Autodesk Fusion 360 part; units mm, degrees
note: some values were not read from the file. Set by a fixed rule: which face or edge a step refers to.
(part 3 of 5)
sketch "Sketch83" plane through (0, 0, 0) normal (0, -1, 0) x (1, 0, 0)
  line L0 (99.6333, 126.9) -> (110.3667, 126.9)
  line L1 (110.3667, 126.9) -> (110.3667, 121.1)
  line L2 (110.3667, 121.1) -> (99.6333, 121.1)
  line L3 (99.6333, 121.1) -> (99.6333, 126.9)
  line L4 (137, 156) -> (105, 156)
  line L5 (105, 156) -> (105, 168)
  line L6 (105, 168) -> (73, 168)
  line L7 (73, 168) -> (73, 134)
  line L8 (99.6333, 134) -> (99.6334, 134)
  line L9 (98.0333, 134) -> (98.0333, 125)
  line L10 (105, 126.9) -> (105, 121.1)
  line L11 (103.9129, 123.9) -> (108.9129, 123.9)
  line L12 (103.9129, 123.9) -> (111.9129, 123.9)
  line L13 (111.9129, 123.9) -> (132.4129, 123.9)
  line L14 (132.4129, 123.9) -> (132.4129, 152.9)
  line L15 (132.4129, 152.9) -> (111.9129, 152.9)
  line L16 (111.9129, 152.9) -> (111.9129, 123.9)
  line L17 (111.9129, 123.9) -> (111.9129, 136.9)
  line L18 (111.9129, 136.9) -> (107.9129, 136.9)
  line L19 (107.9129, 136.9) -> (111.9129, 136.9)
  line L20 (111.9129, 136.9) -> (111.9129, 152.9)
  line L21 (111.9129, 152.9) -> (107.9129, 152.9)
  line L22 (107.9129, 152.9) -> (107.9129, 136.9)
  line L23 (111.9129, 136.9) -> (132.4129, 136.9)
  line L24 (132.4129, 136.9) -> (136.4129, 136.9)
  line L25 (136.4129, 136.9) -> (132.4129, 136.9)
  line L26 (132.4129, 136.9) -> (132.4129, 152.9)
  line L27 (132.4129, 152.9) -> (136.4129, 152.9)
  line L28 (136.4129, 152.9) -> (136.4129, 136.9)
  line L29 (110.3667, 126.9) -> (111.9129, 126.9)
  line L30 (111.9129, 126.9) -> (107.9129, 126.9)
  line L31 (107.9129, 126.9) -> (107.9129, 136.9)
  line L32 (107.9129, 136.9) -> (111.9129, 136.9)
  line L33 (111.9129, 136.9) -> (111.9129, 126.9)
  line L34 (111.9129, 126.9) -> (132.4129, 126.9)
  line L35 (132.4129, 126.9) -> (136.4129, 126.9)
  line L36 (136.4129, 136.9) -> (136.4129, 126.9)
  line L37 (105, 126.9) -> (105, 123.9)
  line L38 (111.9129, 152.9) -> (113.9129, 152.9)
  line L39 (113.9129, 152.9) -> (113.9129, 155)
  line L40 (113.9129, 155) -> (111.9129, 155)
  line L41 (111.9129, 155) -> (111.9129, 152.9)
  line L42 (105, 138.9) -> (105, 133.1)
  line L43 (99.6333, 136) -> (105, 136)
  line L44 (105, 138.9) -> (105, 134)
  line L45 (105, 134) -> (97, 134)
  line L46 (97, 134) -> (76.5, 134)
  line L47 (76.5, 134) -> (76.5, 163)
  line L48 (76.5, 163) -> (97, 163)
  line L49 (97, 163) -> (97, 134)
  line L50 (97, 147) -> (101, 147)
  line L51 (101, 147) -> (97, 147)
  line L52 (97, 147) -> (97, 134)
  line L53 (97, 134) -> (101, 134)
  line L54 (101, 134) -> (101, 147)
  line L55 (97, 147) -> (76.5, 147)
  line L56 (76.5, 147) -> (72.5, 147)
  line L57 (72.5, 147) -> (76.5, 147)
  line L58 (76.5, 147) -> (76.5, 134)
  line L59 (76.5, 134) -> (72.5, 134)
  line L60 (72.5, 134) -> (72.5, 147)
  line L61 (97, 163) -> (95, 163)
  line L62 (95, 163) -> (95, 167)
  line L63 (95, 167) -> (97, 167)
  line L64 (97, 167) -> (97, 163)
  line L65 (97, 167) -> (95, 167)
  line L66 (95, 167) -> (95, 168)
  line L67 (95, 168) -> (97, 168)
  line L68 (97, 168) -> (97, 167)
  line L69 (111.9129, 155) -> (115, 155)
  line L70 (115, 155) -> (115, 156)
  line L71 (115, 156) -> (111.9129, 156)
  line L72 (111.9129, 156) -> (111.9129, 155)
  line L73 (110.3667, 133.1) -> (99.6333, 133.1)
  line L74 (99.6333, 133.1) -> (99.6333, 134)
  line L75 (99.6333, 138.9) -> (110.3667, 138.9)
  line L76 (110.3667, 138.9) -> (110.3667, 133.1)
  line L77 (98.0333, 125) -> (30, 125)
  line L78 (30, 125) -> (30, 115)
  line L79 (30, 115) -> (180, 115)
  line L80 (180, 115) -> (180, 125)
  line L81 (180, 125) -> (137, 125)
  line L82 (137, 125) -> (137, 156)
  line L83 (99.6333, 133.1) -> (105, 133.1)
  line L84 (105, 133.1) -> (105, 138.9)
  line L85 (105, 138.9) -> (99.6333, 138.9)
  line L86 (99.6333, 138.9) -> (99.6333, 133.1)
  line L87 (99.6334, 134) -> (99.6333, 136)
  line L88 (99.6333, 136) -> (99.6333, 138.9)
  line L89 (111.9129, 126.9) -> (107.9129, 126.9)
  line L90 (136.4129, 136.9) -> (137, 136.9)
  line L91 (136.4129, 126.9) -> (137, 126.9)
  line L92 (73, 134) -> (98.0333, 134)
  dimension "d705" = 5
  dimension "d706" = 8
  dimension "d707" = 20.5
  dimension "d708" = 29
  dimension "d709" = 13
  dimension "d710" = 4
  dimension "d711" = 4
  dimension "d712" = 4
  dimension "d715" = 3
  dimension "d716" = 2
  dimension "d718" = 8
  dimension "d719" = 20.5
  dimension "d720" = 29
  dimension "d721" = 4
  dimension "d722" = 13
  dimension "d723" = 4
  dimension "d724" = 2
  dimension "d753" = 2
  constraint midpoint L0 L10.start
  constraint midpoint L2 L10.end
  constraint perpendicular L10 L11
  constraint perpendicular L10 L12
  constraint horizontal L13
  constraint vertical L14
  constraint horizontal L15
  constraint vertical L16
  constraint coincident L16 L17.end
  constraint perpendicular L17 L18
  constraint horizontal L19
  constraint vertical L20
  constraint horizontal L21
  constraint vertical L22
  constraint coincident L14 L23.end
  constraint perpendicular L14 L23
  constraint perpendicular L14 L24
  constraint horizontal L25
  constraint vertical L26
  constraint horizontal L27
  constraint vertical L28
  constraint coincident L0.end L1.start
  constraint coincident L17 L29.end
  constraint horizontal L30
  constraint vertical L31
  constraint horizontal L32
  constraint vertical L33
  constraint coincident L14 L34.end
  constraint perpendicular L14 L34
  constraint perpendicular L35 L36
  constraint perpendicular L11 L37
  constraint coincident L12 L37.end
  constraint horizontal L38
  constraint vertical L39
  constraint horizontal L40
  constraint vertical L41
  constraint midpoint L42 L43.end
  constraint horizontal L46
  constraint vertical L47
  constraint horizontal L48
  constraint vertical L49
  constraint coincident L49 L50.start
  constraint perpendicular L49 L50
  constraint horizontal L51
  constraint vertical L52
  constraint horizontal L53
  constraint vertical L54
  constraint coincident L47 L55.end
  constraint perpendicular L47 L55
  constraint perpendicular L47 L56
  constraint horizontal L57
  constraint vertical L58
  constraint horizontal L59
  constraint vertical L60
  constraint horizontal L61
  constraint vertical L62
  constraint horizontal L63
  constraint vertical L64
  constraint horizontal L65
  constraint vertical L66
  constraint horizontal L67
  constraint vertical L68
  constraint coincident L6 L66.end
  constraint horizontal L69
  constraint vertical L70
  constraint horizontal L71
  constraint vertical L72
  constraint coincident L4 L70.end
  constraint horizontal L83
  constraint vertical L84
  constraint horizontal L85
  constraint vertical L86
  constraint coincident L73.end L74.start
  constraint collinear L29 L30
  constraint coincident L82 L90.end
  constraint perpendicular L82 L90
  constraint coincident L82 L91.end
  constraint perpendicular L82 L91
  measures "d705" distance of L11.start L11.end
  measures "d706" distance of L11.start L12.end
  measures "d707" distance of L12.end L13.end
  measures "d708" distance of L12.end L15.end
  measures "d709" distance of L12.end L17.end
  measures "d710" distance of L17.end L18.end
  measures "d711" distance of L23.end L24.end
  measures "d712" distance of L34.end L35.end
  measures "d715" distance of L10.start L37.end
  measures "d716" distance of L15.end L38.end
  measures "d718" distance of L44.end L45.end
  measures "d719" distance of L45.end L46.end
  measures "d720" distance of L45.end L48.end
  measures "d721" distance of L50.start L50.end
  measures "d722" distance of L45 L50
  measures "d723" distance of L55.end L56.end
  measures "d724" distance of L48.end L61.end
  measures "d753" distance of L43 L45
extrude "Extrude50" cut sketch "Sketch83" against normal blind 10 contours L0 L16 L17 L18 L19 L29 L30 L31 L32 L33 L73 L76 L89 | L1 L12 L16 L17 L29 L30 L89 | L13 L14 L16 L17 L34 | L14 L16 L17 L23 L33 L34 | L14 L15 L16 L20 L23 L26 L38 | L14 L24 L25 L35 L36 | L15 L38 L39 L40 L41 L69 | L36 L82 L90 L91 | L4 L40 L69 L70 L71 L72 bodies 5 in component "inner_adapter"
extrude "Extrude51" cut sketch "Sketch83" against normal blind 10 contours L43 L45 L53 L54 L86 L87 | L45 L49 L50 L51 L52 L53 L54 L75 L85 L86 L87 L88 L92 | L43 L54 L75 L85 L86 L88 | L46 L47 L49 L52 L55 L58 L92 | L47 L48 L49 L55 L61 | L7 L47 L56 L57 L58 L59 L92 | L48 L61 L62 L63 L64 L65 | L7 L56 L57 L59 L60 | L6 L63 L65 L66 L67 L68 bodies 5 in component "inner_adapter"
extrude "Extrude44" add sketch "Sketch81" along normal blind 10 and the other way blind 11 separate body contours L3 L4 L5 L6 L10 | L6 L7 L8 L9 L10 | L25 L27 L37 L40 L41 | L32 L37 L38 L39 L40 makes body 7 at (103.3444, 8, 138.5) makes body 8 at (106.6556, 15, 126.5)
sketch "Sketch84" plane through (100.0333, 0, 0) normal (-1, 0, 0) x (0, -1, 0)
  line L0 (-22, 133.5) -> (-1, 133.5)
  line L1 (-1, 133.5) -> (-1, 138.5)
  line L2 (-1, 138.5) -> (-22, 138.5)
  line L3 (-22, 138.5) -> (-22, 133.5)
  line L4 (-22, 138.5) -> (-16, 138.5)
  line L5 (-22, 133.5) -> (-16, 138.5)
  line L6 (-22, 133.5) -> (-22, 138.5)
  line L7 (-22, 126.5) -> (-22, 121.5)
  line L8 (-22, 121.5) -> (-16, 121.5)
  line L9 (-22, 126.5) -> (-16, 121.5)
  line L10 (0, 125) -> (0, 134)
  line L11 (0, 134) -> (-10, 134)
  line L12 (-10, 134) -> (-11, 134)
  line L13 (-11, 134) -> (-11, 125)
  line L14 (-11, 125) -> (0, 125)
  line L15 (-22, 133.5) -> (-21.5, 133.5)
  line L16 (-21.5, 133.5) -> (-21.5, 133.9167)
  line L17 (-22, 121.5) -> (-1, 121.5)
  line L18 (-22, 126.5) -> (-1, 126.5)
  line L19 (-22, 126.5) -> (-21.5, 126.5)
  line L20 (-21.5, 126.5) -> (-21.5, 126.0833)
  dimension "d731" = 6
  dimension "d732" = 6
  dimension "d948" = 0.5
  dimension "d949" = 0.5
  constraint coincident L2.end L3.start
  constraint perpendicular L3 L4
  constraint coincident L0.start L3.end
  constraint perpendicular L4 L7
  constraint perpendicular L7 L8
  constraint perpendicular L6 L15
  constraint coincident L5 L16.end
  constraint perpendicular L15 L16
  constraint collinear L8 L17
  constraint coincident L7.start L9.start
  constraint perpendicular L7 L19
  constraint coincident L9 L20.end
  constraint perpendicular L19 L20
  measures "d731" distance of L2.end L4.end
  measures "d732" distance of L7.end L8.end
  measures "d948" distance of L0.start L15.end
  measures "d949" distance of L7.start L19.end
extrude "Extrude45" cut sketch "Sketch84" against normal blind 10 contours L0 L5 L15 L16 | L2 L3 L4 L5 L6 | L7 L8 L9 L17 | L9 L18 L19 L20 bodies 8 7
sketch "Sketch85" plane through (100.0333, 0, 0) normal (-1, 0, 0) x (0, -1, 0)
  line L0 (-16, 138.5) -> (-21.5, 133.9167)
  line L1 (-21.5, 133.5) -> (-1, 133.5)
  line L2 (-1, 133.5) -> (-1, 138.5)
  line L3 (-1, 138.5) -> (-16, 138.5)
  line L4 (0, 125) -> (0, 134)
  line L5 (-3, 137.5) -> (-15, 137.5)
  line L6 (-15, 137.5) -> (-15, 134.5)
  line L7 (-15, 134.5) -> (-3, 134.5)
  line L8 (-3, 134.5) -> (-3, 137.5)
  line L9 (-10, 134) -> (-10, 147)
  line L10 (0, 134) -> (-10, 134)
  line L11 (-16, 138.5) -> (-16, 133.5)
  line L12 (-16, 136) -> (-14, 136)
  line L13 (-10, 134) -> (-11, 134)
  line L14 (-11, 134) -> (-11, 125)
  line L15 (-11, 125) -> (0, 125)
  line L16 (-21.5, 133.9167) -> (-21.5, 133.5)
  dimension "d735" = 2
  dimension "d736" = 5
  dimension "d754" = 3
  constraint horizontal L5
  constraint vertical L6
  constraint horizontal L7
  constraint vertical L8
  constraint coincident L0.start L3.end
  constraint coincident L1 L11.end
  constraint perpendicular L1 L11
  constraint midpoint L11 L12.start
  constraint perpendicular L11 L12
  constraint midpoint L6 L12
  measures "d735" distance of L2 L8
  measures "d736" distance of L6 L9
  measures "d754" distance of L5 L7
extrude "Extrude46'" cut sketch "Sketch85" against normal blind 8 contours L5 L6 L7 L9 | L5 L7 L8 L9 bodies 7
copy_body "Body->Comp6" bodies 7 removing the originals makes body 9 in component "Pins"
copy_body "Body->Comp7" bodies 8 removing the originals makes body 10 in component "Component"
copy_body "CutPasteBodies1" bodies 10 removing the originals makes body 11 in component "Pins"
sketch "Sketch86" plane through (0, 0, 0) normal (0, -1, 0) x (1, 0, 0)
  line L0 (97, 168) -> (97, 147)
  line L1 (97, 147) -> (101, 147)
  line L2 (101, 147) -> (101, 138.9)
  line L3 (111.9129, 136.9) -> (111.9129, 156)
  line L4 (111.9129, 156) -> (105, 156)
  line L5 (105, 156) -> (105, 168)
  line L6 (105, 168) -> (97, 168)
  circle A0 centre (105, 143) radius 2
  line L7 (98.0333, 134) -> (98.0333, 125)
  line L8 (132.4129, 126.9) -> (132.4129, 123.9)
  line L9 (132.4129, 123.9) -> (110.3667, 123.9)
  line L10 (110.3667, 123.9) -> (110.3667, 121.1)
  line L11 (110.3667, 121.1) -> (99.6333, 121.1)
  line L12 (99.6333, 121.1) -> (99.6333, 126.9)
  line L13 (99.6333, 126.9) -> (107.9129, 126.9)
  line L14 (101, 138.9) -> (110.3667, 138.9)
  line L15 (110.3667, 138.9) -> (110.3667, 136.9)
  line L16 (99.6333, 134) -> (98.0333, 134)
  line L17 (98.0333, 125) -> (30, 125)
  line L18 (30, 125) -> (30, 115)
  line L19 (30, 115) -> (180, 115)
  line L20 (180, 115) -> (180, 125)
  line L21 (180, 125) -> (137, 125)
  line L22 (137, 125) -> (137, 126.9)
  line L23 (137, 126.9) -> (132.4129, 126.9)
  line L24 (107.9129, 133.1) -> (99.6333, 133.1)
  line L25 (99.6333, 133.1) -> (99.6333, 134)
  line L26 (110.3667, 136.9) -> (111.9129, 136.9)
  line L27 (107.9129, 126.9) -> (107.9129, 133.1)
  circle A1 centre (101, 164) radius 2
  dimension "d740" = 4
  dimension "d929" = 4
  dimension "d930" = 4
  dimension "d931" = 4
  measures "d740" diameter of A0
  measures "d929" diameter of A1
  measures "d930" distance of L6 A1.centre
  measures "d931" distance of L0 A1.centre
extrude "Extrude52" cut sketch "Sketch86" against normal blind 8 contours A0 | A1 bodies 5 in component "inner_adapter"
sketch "Sketch87" plane through (101, 0, 0) normal (-1, 0, 0) x (0, -1, 0)
  line L0 (0, 138.9) -> (0, 147)
  line L1 (0, 147) -> (-10, 147)
  line L2 (-10, 147) -> (-10, 138.9)
  line L3 (-8, 145) -> (-8, 141)
  line L4 (0, 145) -> (0, 141)
  line L5 (-8, 146.5) -> (-4.9, 146.5)
  line L6 (-4.9, 146.5) -> (-4.9, 139.5)
  line L7 (-4.9, 139.5) -> (-8, 139.5)
  line L8 (-8, 139.5) -> (-8, 146.5)
  line L9 (-10, 138.9) -> (0, 138.9)
  dimension "d745" = 3.1
  dimension "d746" = 7
  constraint horizontal L5
  constraint vertical L6
  constraint horizontal L7
  constraint vertical L8
  constraint midpoint L3 L8
  measures "d745" distance of L5.start L5.end
  measures "d746" distance of L5.start L7.end
sketch "Sketch102" plane through (105, 0, 0) normal (1, 0, 0) x (0, 1, 0)
  line L0 (11, 156) -> (11, 168)
  line L1 (11, 168) -> (0, 168)
  line L2 (0, 168) -> (0, 156)
  line L3 (0, 156) -> (11, 156)
  line L4 (8, 162) -> (8, 166)
  line L5 (0, 162) -> (0, 166)
  line L6 (8, 164) -> (8, 160.5)
  line L7 (8, 160.5) -> (4.9, 160.5)
  line L8 (4.9, 160.5) -> (4.9, 167.5)
  line L9 (4.9, 167.5) -> (8, 167.5)
  line L10 (8, 167.5) -> (8, 160.5)
  dimension "d932" = 3.5
  dimension "d933" = 3.1
  dimension "d934" = 7
  constraint midpoint L4 L6.start
  constraint parallel L4 L6
  constraint horizontal L7
  constraint vertical L8
  constraint horizontal L9
  constraint vertical L10
  measures "d932" distance of L6.start L6.end
  measures "d933" distance of L6.end L7.end
  measures "d934" distance of L6.end L9.end
extrude "Extrude60" cut sketch "Sketch102" against normal blind 8 contours L4 L6 L7 L8 L9 L10 bodies 5 in component "inner_adapter"
extrude "Extrude53" cut sketch "Sketch87" against normal blind 8 contours L3 L5 L6 L7 L8 bodies 5 in component "inner_adapter"
sketch "Sketch89" plane through (109.9667, 0, 0) normal (1, 0, 0) x (0, 1, 0)
  line L0 (16, 121.5) -> (21.5, 126.0833)
  line L1 (21.5, 126.5) -> (1, 126.5)
  line L2 (1, 126.5) -> (1, 121.5)
  line L3 (1, 121.5) -> (16, 121.5)
  line L4 (16, 121.5) -> (16, 126.5)
  line L5 (16, 124) -> (14, 124)
  line L6 (3, 125.5) -> (15, 125.5)
  line L7 (15, 125.5) -> (15, 122.5)
  line L8 (15, 122.5) -> (3, 122.5)
  line L9 (3, 122.5) -> (3, 125.5)
  line L10 (3, 134.5) -> (3, 137.5)
  line L11 (3, 137.5) -> (15, 137.5)
  line L12 (15, 137.5) -> (15, 134.5)
  line L13 (15, 134.5) -> (3, 134.5)
  line L14 (3, 137.5) -> (3, 121.5)
  line L15 (15, 137.5) -> (15, 121)
  line L16 (21.5, 126.0833) -> (21.5, 126.5)
  dimension "d758" = 3
  constraint coincident L0.start L3.end
  constraint coincident L1 L4.end
  constraint perpendicular L1 L4
  constraint midpoint L4 L5.start
  constraint perpendicular L4 L5
  constraint horizontal L6
  constraint vertical L7
  constraint horizontal L8
  constraint vertical L9
  constraint midpoint L5 L7
  constraint coincident L10.end L11.start
  constraint perpendicular L11 L14
  constraint coincident L11.end L12.start
  constraint perpendicular L11 L15
  constraint collinear L7 L15
  constraint collinear L9 L14
  measures "d758" distance of L6 L8
extrude "Extrude1'''" cut sketch "Sketch89" against normal blind 8 contours L6 L7 L8 L9 L14 L15 bodies 11 in component "Pins"
sketch "Sketch126" plane through (0, 16, 0) normal (0, 1, 0) x (-1, 0, 0)
  line L0 (-135, 115) -> (-75, 115)
  line L1 (-75, 115) -> (-75, 205)
  line L2 (-75, 205) -> (-135, 205)
  line L3 (-135, 205) -> (-135, 115)
  line L4 (-110.3667, 138.9) -> (-99.6333, 138.9)
  line L5 (-99.6333, 138.9) -> (-99.6333, 133.1)
  line L6 (-99.6333, 133.1) -> (-110.3667, 133.1)
  line L7 (-110.3667, 133.1) -> (-110.3667, 138.9)
  line L8 (-110.3667, 121.1) -> (-110.3667, 126.9)
  line L9 (-110.3667, 126.9) -> (-99.6333, 126.9)
  line L10 (-99.6333, 126.9) -> (-99.6333, 121.1)
  line L11 (-99.6333, 121.1) -> (-110.3667, 121.1)
  line L12 (-115, 131.5) -> (-95, 131.5)
  line L13 (-95, 131.5) -> (-95, 128.5)
  line L14 (-95, 128.5) -> (-115, 128.5)
  line L15 (-115, 128.5) -> (-115, 131.5)
  line L16 (-105, 126.9) -> (-105, 128.5)
  dimension "d1103" = 20
  dimension "d1104" = 3
  dimension "d1105" = 1.6
  constraint horizontal L12
  constraint vertical L13
  constraint horizontal L14
  constraint vertical L15
  constraint midpoint L9 L16.start
  constraint midpoint L14 L16.end
  constraint parallel L8 L16
  measures "d1103" distance of L12.start L12.end
  measures "d1104" distance of L12.start L14.end
  measures "d1105" distance of L16.start L16.end
extrude "Extrude77" cut sketch "Sketch126" against normal blind 3 contours L12 L13 L14 L15 bodies 5 in component "inner_adapter"
sketch "Sketch127" plane through (0, 18, 0) normal (0, -1, 0) x (1, 0, 0)
  line L0 (75, 127.5) -> (135, 127.5)
  line L1 (135, 127.5) -> (135, 132.5)
  line L2 (135, 132.5) -> (75, 132.5)
  line L3 (75, 132.5) -> (75, 127.5)
  line L4 (95, 131.5) -> (115, 131.5)
  line L5 (115, 131.5) -> (95, 131.5)
  line L6 (115, 131.5) -> (95, 131.5)
  line L7 (95, 128.5) -> (115, 128.5)
  line L8 (95, 131.5) -> (95, 128.5)
  line L9 (115, 128.5) -> (115, 131.5)
extrude "Extrude10" cut sketch "Sketch127" against normal blind 3 contours L4 L5 L6 L7 L8 L9 bodies 6 in component "Flap"
sketch "Sketch95" plane through (0, 0, 0) normal (0, -1, 0) x (1, 0, 0)
  circle A0 centre (105, 143) radius 2
  line L0 (97, 168) -> (97, 147)
  line L1 (97, 147) -> (101, 147)
  line L2 (101, 147) -> (101, 138.9)
  line L3 (111.9129, 136.9) -> (111.9129, 156)
  line L4 (111.9129, 156) -> (105, 156)
  line L5 (105, 156) -> (105, 168)
  line L6 (105, 168) -> (97, 168)
  line L7 (95, 163) -> (95, 168)
  line L8 (95, 168) -> (73, 168)
  line L9 (73, 168) -> (73, 147)
  line L10 (73, 147) -> (76.5, 147)
  line L11 (76.5, 147) -> (76.5, 163)
  line L12 (76.5, 163) -> (95, 163)
  line L13 (98.0333, 134) -> (98.0333, 125)
  line L14 (132.4129, 126.9) -> (132.4129, 123.9)
  line L15 (132.4129, 123.9) -> (110.3667, 123.9)
  line L16 (110.3667, 123.9) -> (110.3667, 121.1)
  line L17 (110.3667, 121.1) -> (99.6333, 121.1)
  line L18 (99.6333, 121.1) -> (99.6333, 126.9)
  line L19 (99.6333, 126.9) -> (107.9129, 126.9)
  line L20 (73, 168) -> (137, 168)
  line L21 (137, 168) -> (137, 125)
  line L22 (137, 125) -> (73, 125)
  line L23 (73, 125) -> (73, 168)
  circle A1 centre (105, 143) radius 2
  line L24 (110.3667, 138.9) -> (110.3667, 136.9)
  line L25 (101, 138.9) -> (110.3667, 138.9)
  line L26 (110.3667, 123.9) -> (110.3667, 126.9)
  line L27 (110.3667, 138.9) -> (94.3667, 138.9)
  line L28 (94.3667, 138.9) -> (94.3667, 133.1)
  line L29 (94.3667, 133.1) -> (110.3667, 133.1)
  line L30 (110.3667, 133.1) -> (110.3667, 138.9)
  line L31 (110.3667, 126.9) -> (99.6333, 126.9)
  line L32 (99.6333, 126.9) -> (99.6333, 121.1)
  line L33 (99.6333, 121.1) -> (110.3667, 121.1)
  line L34 (110.3667, 121.1) -> (110.3667, 126.9)
  line L35 (137, 125) -> (99.6333, 125)
  line L36 (99.6333, 125) -> (99.6333, 121.1)
  line L37 (99.6333, 121.1) -> (137, 121.1)
  line L38 (137, 121.1) -> (137, 125)
  line L39 (137, 121.1) -> (73, 121.1)
  line L40 (73, 121.1) -> (73, 125)
  line L41 (73, 125) -> (137, 125)
  line L42 (137, 125) -> (137, 121.1)
  line L43 (73, 121.1) -> (137, 121.1)
  line L44 (137, 121.1) -> (137, 118.1)
  line L45 (137, 118.1) -> (73, 118.1)
  line L46 (73, 118.1) -> (73, 121.1)
  line L47 (101, 138.9) -> (110.3667, 138.9)
  line L48 (110.3667, 138.9) -> (110.3667, 136.9)
  line L49 (99.6333, 134) -> (98.0333, 134)
  line L50 (98.0333, 125) -> (30, 125)
  line L51 (30, 125) -> (30, 115)
  line L52 (30, 115) -> (180, 115)
  line L53 (180, 115) -> (180, 125)
  line L54 (180, 125) -> (137, 125)
  line L55 (137, 125) -> (137, 126.9)
  line L56 (137, 126.9) -> (132.4129, 126.9)
  line L57 (107.9129, 133.1) -> (99.6333, 133.1)
  line L58 (99.6333, 133.1) -> (99.6333, 134)
  line L59 (137, 126.9) -> (132.4129, 126.9)
  line L60 (110.3667, 136.9) -> (111.9129, 136.9)
  line L61 (107.9129, 126.9) -> (107.9129, 133.1)
  circle A2 centre (101, 164) radius 2
  line L62 (99.6333, 126.9) -> (115.6333, 126.9)
  line L63 (115.6333, 126.9) -> (115.6333, 121.1)
  line L64 (115.6333, 121.1) -> (99.6333, 121.1)
  line L65 (99.6333, 121.1) -> (99.6333, 126.9)
  line L66 (95, 168) -> (95, 170)
  line L67 (95, 170) -> (71, 170)
  line L68 (71, 170) -> (71, 147)
  line L69 (71, 147) -> (73, 147)
  line L70 (137, 156) -> (115, 156)
  line L71 (137, 156) -> (115, 156)
  line L72 (115, 156) -> (115, 158)
  line L73 (115, 158) -> (137, 158)
  line L74 (137, 158) -> (137, 156)
  line L75 (137, 158) -> (139, 158)
  line L76 (139, 158) -> (139, 125)
  line L77 (93.8667, 132.6) -> (110.8667, 132.6)
  line L78 (110.8667, 132.6) -> (110.8667, 139.4)
  line L79 (110.8667, 139.4) -> (93.8667, 139.4)
  line L80 (93.8667, 139.4) -> (93.8667, 132.6)
  line L81 (99.1333, 127.4) -> (116.1333, 127.4)
  line L82 (116.1333, 127.4) -> (116.1333, 120.6)
  line L83 (116.1333, 120.6) -> (99.1333, 120.6)
  line L84 (99.1333, 120.6) -> (99.1333, 127.4)
  point P0 (107.9129, 126.9)
  dimension "d873" = 3
  dimension "d945" = 16
  dimension "d946" = 16
  dimension "d969" = 2
  dimension "d970" = 24
  dimension "d971" = 2
  dimension "d972" = 2
  dimension "d977" = 2
  dimension "d1044" = 0.5
  dimension "d1045" = -0.5
  constraint horizontal L20
  constraint vertical L21
  constraint horizontal L22
  constraint vertical L23
  constraint coincident L8.end L9.start
  constraint horizontal L27
  constraint vertical L28
  constraint horizontal L29
  constraint vertical L30
  constraint coincident L24.start L25.end
  constraint horizontal L31
  constraint vertical L32
  constraint horizontal L33
  constraint vertical L34
  constraint coincident L17.end L18.start
  constraint coincident L26.end L31.start
  constraint horizontal L35
  constraint vertical L36
  constraint horizontal L37
  constraint vertical L38
  constraint horizontal L39
  constraint vertical L40
  constraint horizontal L41
  constraint vertical L42
  constraint horizontal L43
  constraint vertical L44
  constraint horizontal L45
  constraint vertical L46
  constraint horizontal L62
  constraint vertical L63
  constraint horizontal L64
  constraint vertical L65
  constraint coincident L7.end L8.start
  constraint perpendicular L8 L66
  constraint perpendicular L66 L67
  constraint perpendicular L67 L68
  constraint perpendicular L23 L69
  constraint horizontal L71
  constraint vertical L72
  constraint horizontal L73
  constraint vertical L74
  constraint coincident L70.start L71.start
  constraint perpendicular L21 L75
  constraint coincident L54 L76.end
  constraint perpendicular L54 L76
  measures "d873" distance of L39.end L45.end
  measures "d945" distance of L24.start L27.end
  measures "d946" distance of L18.end L62.end
  measures "d969" distance of L7.end L66.end
  measures "d970" distance of L66.end L67.end
  measures "d971" distance of L68.end L9.end
  measures "d972" distance of L70.start L73.end
  measures "d977" distance of L73.end L75.end
extrude "Extrude47'" add sketch "Sketch95" along normal blind 5 separate body contours L0 L1 L2 L3 L4 L5 L6 L20 L60 L78 L79 | L0 L1 L2 L7 L10 L11 L12 L13 L20 L22 L23 L41 L50 L77 L79 L80 | L3 L4 L5 L14 L20 L21 L22 L35 L41 L56 L59 L60 L61 L70 L71 L72 L73 L77 L78 L81 L82 | L7 L8 L9 L10 L11 L12 L20 L23 | L8 L9 L20 L23 L66 L67 L68 L69 | L21 L54 L55 L74 L75 L76 | L21 L70 L71 L72 L73 L74 | L22 L39 L40 L41 L43 L50 L84 | L14 L21 L22 L35 L41 L55 L56 L59 | L13 L22 L41 L61 L77 L81 L84 | L37 L39 L43 L44 L45 L46 L82 L83 L84 | L14 L15 L22 L35 L37 L38 L39 L41 L42 L43 L82 | L14 L15 L22 L35 L41 L82 makes body 12
extrude "Extrude59'" add sketch "Sketch95" against normal blind 11 contours L8 L9 L20 L23 L66 L67 L68 L69 | L21 L54 L55 L74 L75 L76 | L21 L70 L71 L72 L73 L74 bodies 12
sketch "Sketch96" plane through (0, -5, 0) normal (0, -1, 0) x (1, 0, 0)
  circle A0 centre (105, 143) radius 2
  line L0 (73, 118.1) -> (137, 118.1)
  line L1 (137, 118.1) -> (137, 125)
  line L2 (137, 168) -> (95, 168)
  line L3 (73, 147) -> (73, 118.1)
  line L4 (94.3667, 138.9) -> (94.3667, 139.9)
  line L5 (94.3667, 139.9) -> (93.3667, 139.9)
  line L6 (115.6333, 121.1) -> (116.6333, 121.1017)
  line L7 (116.6333, 121.1017) -> (116.6351, 120.1017)
  line L8 (116.6351, 120.1017) -> (93.3667, 120.1017)
  line L9 (93.3667, 120.1017) -> (93.3667, 139.9)
  line L10 (93.3667, 139.9) -> (116.6351, 139.9)
  line L11 (116.6351, 139.9) -> (116.6351, 120.1017)
  line L12 (94.3667, 133.1) -> (94.3667, 132.1)
  line L13 (115.6333, 126.9) -> (115.6333, 127.9)
  line L14 (116.6351, 127.9) -> (93.3667, 127.9)
  line L15 (93.3667, 132.1) -> (116.6351, 132.1)
  circle A1 centre (105.0009, 136) radius 2.1
  line L16 (105.0009, 139.9) -> (105.0009, 132.1)
  line L17 (105.0009, 127.9) -> (105.0009, 120.1017)
  circle A2 centre (105.0009, 124.0009) radius 2.1
  circle A3 centre (101, 164) radius 2
  line L18 (95, 168) -> (95, 170)
  line L19 (95, 170) -> (71, 170)
  line L20 (71, 170) -> (71, 147)
  line L21 (71, 147) -> (73, 147)
  line L22 (137, 125) -> (139, 125)
  line L23 (139, 125) -> (139, 158)
  line L24 (139, 158) -> (137, 158)
  line L25 (137, 158) -> (137, 168)
  line L26 (93.8667, 132.6) -> (93.8667, 139.4)
  line L27 (93.8667, 139.4) -> (110.8667, 139.4)
  line L28 (110.8667, 139.4) -> (110.8667, 132.6)
  line L29 (110.8667, 132.6) -> (93.8667, 132.6)
  line L30 (116.1333, 120.6) -> (99.1333, 120.6)
  line L31 (99.1333, 120.6) -> (99.1333, 127.4)
  line L32 (99.1333, 127.4) -> (116.1333, 127.4)
  line L33 (116.1333, 127.4) -> (116.1333, 120.6)
  dimension "d876" = 1
  dimension "d877" = 1
  dimension "d878" = 1
  dimension "d879" = 1
  dimension "d880" = 1
  dimension "d881" = 1
  dimension "d882" = 4.2
  dimension "d883" = 4.2
  constraint perpendicular L4 L5
  constraint perpendicular L6 L7
  constraint horizontal L8
  constraint vertical L9
  constraint horizontal L10
  constraint vertical L11
  constraint coincident L11 L14.start
  constraint coincident L9 L14.end
  constraint perpendicular L9 L14
  constraint coincident L9 L15.start
  constraint coincident L11 L15.end
  constraint perpendicular L11 L15
  constraint coincident L12.end L15
  constraint coincident L13.end L14
  constraint midpoint L10 L16.start
  constraint midpoint L15 L16.end
  constraint midpoint A1.centre L16
  constraint midpoint L14 L17.start
  constraint midpoint L8 L17.end
  constraint midpoint L17 A2.centre
  measures "d876" distance of L4.start L4.end
  measures "d877" distance of L4.end L5.end
  measures "d878" distance of L6.start L6.end
  measures "d879" distance of L6.end L7.end
  measures "d880" distance of L12.start L12.end
  measures "d881" distance of L13.start L13.end
  measures "d882" diameter of A1
  measures "d883" diameter of A2
extrude "Extrude48'" add sketch "Sketch96" along normal blind 9 contours L4 L5 L9 L10 L12 L15 L26 L27 L29 | A1 L16 L26 L27 L29 | L4 L10 L16 L27 | A1 L16 L27 L28 L29 | L10 L11 L15 L16 L27 L28 L29 | L9 L11 L14 L15 | L12 L15 L16 L29 | L8 L9 L14 L17 L30 L31 L32 | L13 L14 L17 L32 | L6 L11 L13 L14 L32 L33 | L6 L7 L8 L11 L17 L30 L33 | L17 A2 L30 L32 L33 | L17 A2 L30 L31 L32 bodies 12
extrude "Extrude49'" add sketch "Sketch96" along normal blind 2 from surface at 9 contours L4 L5 L9 L10 L12 L15 L26 L27 L29 | A1 L16 L26 L27 L29 | L4 L10 L16 L27 | A1 L16 L27 L28 L29 | L10 L11 L15 L16 L27 L28 L29 | A1 L16 | A1 L16 | L9 L11 L14 L15 | L12 L15 L16 L29 | L8 L9 L14 L17 L30 L31 L32 | L13 L14 L17 L32 | L6 L11 L13 L14 L32 L33 | L6 L7 L8 L11 L17 L30 L33 | L17 A2 L30 L32 L33 | L17 A2 L30 L31 L32 | L17 A2 | L17 A2 bodies 12
copy_body "Body->Comp8" bodies 12 removing the originals makes body 13 in component "Mechanism_backstop"
sketch "Skizze97" plane through (0, 0, 125) normal (0, 0, 1) x (-1, 0, 0)
  line L0 (-21.3369, -104.8) -> (-24.8369, -104.8)
  line L1 (-24.8369, -104.8) -> (-24.8369, -99.2)
  line L2 (-24.8369, -99.2) -> (-21.3369, -99.2)
  line L3 (-21.3369, -99.2) -> (-21.3369, -104.8)
  line L4 (-185.1631, -104.8) -> (-188.6631, -104.8)
  line L5 (-188.6631, -104.8) -> (-188.6631, -99.2)
  line L6 (-188.6631, -99.2) -> (-185.1631, -99.2)
  line L7 (-185.1631, -99.2) -> (-185.1631, -104.8)
  circle A0 centre (-11, -70) radius 2
  circle A1 centre (-199, -70) radius 2
  circle A2 centre (-11, -140) radius 2
  circle A3 centre (-199, -140) radius 2
  circle A4 centre (-199, -35) radius 3.5
  circle A5 centre (-11, -35) radius 3.5
  circle A6 centre (-199, -175) radius 3.5
  circle A7 centre (-11, -175) radius 3.5
  arc A8 (-180, 0) -> (-210, -30) centre (-180, -30) ccw
  line L8 (-210, -30) -> (-210, -180)
  arc A9 (-210, -180) -> (-180, -210) centre (-180, -180) ccw
  line L9 (-180, -210) -> (-30, -210)
  arc A10 (-30, -210) -> (0, -180) centre (-30, -180) ccw
  line L10 (0, -180) -> (0, -30)
  arc A11 (0, -30) -> (-30, 0) centre (-30, -30) ccw
  line L11 (-137, 0) -> (-180, 0)
  line L12 (-98.0333, -11) -> (-75, -11)
  spline S0 degree 3 poles (-75, -11) (-73.6669, -11) (-72.3215, -11.1868) (-70.7827, -11.5209) (-69.7039, -11.7551) (-68.5449, -12.0678) (-67.3101, -12.4666) (-63.5716, -13.6741) (-59.3264, -15.5672) (-54.921, -17.8316) (-52.6617, -18.993) (-50.3688, -20.252) (-48.1137, -21.5656) (-43.134, -24.4661) (-38.3659, -27.5905) (-34.4467, -30.5403) (-31.6285, -32.6614) (-29.2725, -34.6734) (-27.4088, -36.5974) (-26.9392, -37.0821) (-26.4696, -37.5669) (-26, -38.0516) knots 0 0 0 0 0.068385 0.068385 0.068385 0.116327 0.116327 0.116327 0.262353 0.262353 0.262353 0.337245 0.337245 0.337245 0.502934 0.502934 0.502934 0.621914 0.621914 0.621914 0.656812 0.656812 0.656812 0.656812
  line L13 (-26, -38.0516) -> (-26, -157.5)
  line L14 (-26, -157.5) -> (-12.5, -157.5)
  line L15 (-18, -160.5) -> (-18, -186.5)
  line L16 (-18, -186.5) -> (-25, -186.5)
  line L17 (-25, -186.5) -> (-25, -160.5)
  line L18 (-26, -183) -> (-101.02, -183)
  ellipse E0 centre (-105, -188.2858) end of major axis (-105, -180.5592) minor radius 5.4567 (-108.98, -183) -> (-101.02, -183) ccw
  line L19 (-184, -183) -> (-184, -160.5)
  line L20 (-185, -160.5) -> (-185, -186.5)
  line L21 (-185, -186.5) -> (-192, -186.5)
  line L22 (-192, -186.5) -> (-192, -160.5)
  spline S1 degree 3 poles (-184, -38.0508) (-183.53, -37.5659) (-183.0599, -37.0811) (-182.5899, -36.5963) (-180.4883, -34.4285) (-177.7611, -32.1455) (-174.4691, -29.7357) (-169.3238, -25.9693) (-162.8741, -21.9475) (-156.519, -18.5779) (-152.2041, -16.29) (-147.9761, -14.3309) (-144.2124, -12.9853) (-141.9329, -12.1703) (-139.8769, -11.6068) (-138.0391, -11.287) (-137.6862, -11.2256) (-137.3408, -11.1732) (-137, -11.1307) knots -0.65681 -0.65681 -0.65681 -0.65681 -0.621923 -0.621923 -0.621923 -0.48793 -0.48793 -0.48793 -0.278155 -0.278155 -0.278155 -0.135918 -0.135918 -0.135918 -0.050335 -0.050335 -0.050335 -0.033901 -0.033901 -0.033901 -0.033901
  line L23 (-116.6351, 5) -> (-93.3667, 5)
  line L24 (-93.3667, 5) -> (-93.3667, 16)
  line L25 (-93.3667, 16) -> (-116.6351, 16)
  line L26 (-116.6351, 16) -> (-116.6351, 5)
  line L27 (-137, 0) -> (-95, 0)
  line L28 (-95, 5) -> (-137, 5)
  line L29 (-137, 5) -> (-137, 0)
  arc A12 (-180, -5) -> (-205, -30) centre (-180, -30) ccw
  line L30 (-205, -30) -> (-205, -180)
  arc A13 (-205, -180) -> (-180, -205) centre (-180, -180) ccw
  line L31 (-180, -205) -> (-30, -205)
  arc A14 (-30, -205) -> (-5, -180) centre (-30, -180) ccw
  line L32 (-5, -180) -> (-5, -30)
  arc A15 (-5, -30) -> (-30, -5) centre (-30, -30) ccw
  line L33 (-93.3667, 18) -> (-116.6351, 18)
  line L34 (-116.6351, 18) -> (-180, -5)
  line L35 (-93.3667, 18) -> (-30, -5)
  line L36 (-93.3667, 23) -> (-116.6351, 23)
  line L37 (-116.6351, 23) -> (-180, 0)
  line L38 (-180, -210) -> (-30, -210)
  arc A16 (-30, -210) -> (0, -180) centre (-30, -180) ccw
  line L39 (0, -180) -> (0, -30)
  arc A17 (0, -30) -> (-30, 0) centre (-30, -30) ccw
  arc A18 (-180, 0) -> (-210, -30) centre (-180, -30) ccw
  line L40 (-210, -30) -> (-210, -180)
  arc A19 (-210, -180) -> (-180, -210) centre (-180, -180) ccw
  line L41 (-199, -140) -> (-190, -140)
  line L42 (-199, -140) -> (-199, -150)
  line L43 (-199, -150) -> (-205, -150)
  line L44 (-199, -70) -> (-190, -70)
  line L45 (-199, -70) -> (-199, -50)
  line L46 (-199, -50) -> (-205, -50)
  line L47 (-190, -140) -> (-190, -70)
  line L48 (-105, -191.1402) -> (-105, -26.9364)
  line L49 (-199, -150) -> (-190, -150)
  line L50 (-190, -150) -> (-190, -140)
  line L51 (-190, -140) -> (-199, -140)
  line L52 (-199, -140) -> (-199, -150)
  line L53 (-199, -145) -> (-205, -145)
  line L54 (-199, -145) -> (-195, -145)
  line L55 (-195, -145) -> (-195, -140)
  line L56 (-195, -140) -> (-195, -71.0732)
  line L57 (-202.2329, -55) -> (-205, -55)
  line L58 (-11, -150) -> (-5, -150)
  line L59 (-11, -150) -> (-20, -150)
  line L60 (-11, -145) -> (-5, -145)
  line L61 (-11, -145) -> (-15, -145)
  line L62 (-15, -145) -> (-15, -140)
  line L63 (-20, -150) -> (-20, -140)
  line L64 (-15, -140) -> (-15, -71.0732)
  line L65 (-20, -140) -> (-20, -70)
  line L66 (-7.7671, -55) -> (-5, -55)
  line L67 (-11, -50) -> (-5, -50)
  line L68 (-205, -145) -> (-210, -145)
  line L69 (-205, -55) -> (-210, -55)
  line L70 (-5, -55) -> (0, -55)
  line L71 (-5, -145) -> (0, -145)
  line L72 (-20, -70) -> (-20, -50)
  line L73 (-20, -50) -> (-11, -50)
  line L74 (-15, -71.0732) -> (-15, -55)
  line L75 (-15, -55) -> (-7.7671, -55)
  line L76 (-190, -50) -> (-199, -50)
  line L77 (-195, -55) -> (-202.2329, -55)
  line L78 (-195, -71.0732) -> (-195, -55)
  line L79 (-190, -70) -> (-190, -50)
  line L80 (-137, -11.1307) -> (-137, 0)
  line L81 (-98.0333, 0) -> (-98.0333, -11)
  line L82 (-197.5, -157.5) -> (-184, -157.5)
  line L83 (-184, -157.5) -> (-184, -38.0508)
  line L84 (-93.3667, 23) -> (-30, 0)
  line L85 (-95, 0) -> (-95, 5)
  line L86 (-108.98, -183) -> (-184, -183)
  line L87 (-12.5, -157.5) -> (-12.5, -162.5)
  line L88 (-197.5, -162.5) -> (-197.5, -157.5)
  line L89 (-196.5, -162.5) -> (-197.5, -162.5)
  line L90 (-13.5, -160.5) -> (-18, -160.5)
  line L91 (-26, -160.5) -> (-26, -183)
  line L92 (-184, -160.5) -> (-185, -160.5)
  line L93 (-12.5, -162.5) -> (-13.5, -162.5)
  line L94 (-13.5, -162.5) -> (-13.5, -160.5)
  line L95 (-25, -160.5) -> (-26, -160.5)
  line L96 (-192, -160.5) -> (-196.5, -160.5)
  line L97 (-196.5, -160.5) -> (-196.5, -162.5)
  line L98 (-30, 0) -> (-98.0333, 0)
  dimension "d889" = -5
  dimension "d890" = 2
  dimension "d891" = 7
  dimension "d892" = 9
  dimension "d893" = 10
  dimension "d894" = 9
  dimension "d895" = 20
  constraint coincident A8.start L11.end
  constraint coincident A3.centre L41.start
  constraint horizontal L41
  constraint perpendicular L41 L42
  constraint coincident L30 L43.end
  constraint perpendicular L30 L43
  constraint coincident A1.centre L44.start
  constraint horizontal L44
  constraint perpendicular L44 L45
  constraint coincident L30 L46.end
  constraint perpendicular L30 L46
  constraint horizontal L49
  constraint vertical L50
  constraint horizontal L51
  constraint vertical L52
  constraint symmetric L41.end L48 L63.end
  constraint symmetric L42.end L48 L58.start
  constraint symmetric L43.end L48 L58.end
  constraint symmetric L44.end L48 L65.end
  constraint symmetric L45.end L48 L67.start
  constraint symmetric L46.end L48 L67.end
  constraint symmetric L48 L49.end L59.end
  constraint symmetric L48 L53.start L60.start
  constraint symmetric L48 L53.end L60.end
  constraint symmetric L48 L54.end L61.end
  constraint symmetric L48 L55.end L62.end
  constraint symmetric L48 L56.end L64.end
  constraint symmetric L48 L57.start L66.start
  constraint symmetric L48 L57.end L66.end
  constraint perpendicular L30 L68
  constraint coincident L8 L69.end
  constraint perpendicular L8 L69
  constraint coincident L39 L70.end
  constraint perpendicular L39 L70
  constraint coincident L10 L71.end
  constraint perpendicular L10 L71
  constraint perpendicular L67 L72
  constraint perpendicular L32 L73
  constraint parallel L64 L74
  constraint symmetric L48 L64.end L56.end
  constraint symmetric L48 L65.end L44.end
  constraint symmetric L48 L66.start L57.start
  constraint symmetric L48 L67.start L45.end
  constraint symmetric L48 L72.end L76.start
  constraint symmetric L48 L74.end L77.start
  constraint coincident A11.end A17.end
  measures "d892" distance of A3.centre L41.end
  measures "d893" distance of A3.centre L42.end
  measures "d894" distance of A1.centre L44.end
  measures "d895" distance of A1.centre L45.end
sketch "Sketch103" plane through (0, 1, 0) normal (0, -1, 0) x (1, 0, 0)
  line L0 (109.9667, 133.5) -> (109.9667, 138.5)
  line L1 (109.9667, 138.5) -> (100.0333, 138.5)
  line L2 (100.0333, 138.5) -> (100.0333, 133.5)
  line L3 (100.0333, 133.5) -> (109.9667, 133.5)
  circle A0 centre (105, 136) radius 2
  dimension "d939" = 4
  measures "d939" diameter of A0
extrude "Extrude2'" cut sketch "Sketch103" against normal blind 1 contours A0 bodies 9 in component "Pins"
sketch "Sketch104" plane through (0, 1, 0) normal (0, -1, 0) x (1, 0, 0)
  line L0 (109.9667, 121.5) -> (109.9667, 126.5)
  line L1 (109.9667, 126.5) -> (100.0333, 126.5)
  line L2 (100.0333, 126.5) -> (100.0333, 121.5)
  line L3 (100.0333, 121.5) -> (109.9667, 121.5)
  circle A0 centre (105, 124) radius 2
  dimension "d942" = 4
  measures "d942" diameter of A0
extrude "Extrude3''" cut sketch "Sketch104" against normal blind 1 contours A0 bodies 11 in component "Pins"
sketch "Sketch105" plane through (0, 0, 139.4) normal (0, 0, -1) x (1, 0, 0)
  line L0 (93.8667, 0) -> (88.8667, 0)
  line L1 (88.8667, 0) -> (93.8667, 5)
  line L2 (93.8667, 0) -> (110.8667, 0)
  line L3 (110.8667, 0) -> (110.8667, 5)
  line L4 (110.8667, 5) -> (93.8667, 5)
  line L5 (93.8667, 5) -> (93.8667, 0)
  line L6 (93.8667, 0) -> (110.8667, 0)
  line L7 (110.8667, 0) -> (110.8667, 5)
  line L8 (110.8667, 5) -> (93.8667, 5)
  line L9 (93.8667, 5) -> (93.8667, 0)
  dimension "d950" = 5
  constraint horizontal L0
  constraint coincident L0.start L2.start
  constraint coincident L1.end L4.end
  measures "d950" distance of L0.start L0.end
extrude "Extrude1''''" cut sketch "Sketch105" along normal up to surface (6.8 mm away) contours L0 L1 L5 L9 bodies 13 in component "Mechanism_backstop"
sketch "Sketch106" plane through (0, 0, 127.4) normal (0, 0, -1) x (1, 0, 0)
  line L0 (116.1333, 0) -> (121.1333, 0)
  line L1 (121.1333, 0) -> (116.1333, 5)
  line L2 (99.1333, 0) -> (116.1333, 0)
  line L3 (116.1333, 0) -> (116.1333, 5)
  line L4 (116.1333, 5) -> (99.1333, 5)
  line L5 (99.1333, 5) -> (99.1333, 0)
  line L6 (99.1333, 0) -> (116.1333, 0)
  line L7 (116.1333, 0) -> (116.1333, 5)
  line L8 (116.1333, 5) -> (99.1333, 5)
  line L9 (99.1333, 5) -> (99.1333, 0)
  dimension "d954" = 5
  constraint horizontal L0
  constraint coincident L0.start L2.end
  constraint coincident L1.end L3.end
  measures "d954" distance of L0.start L0.end
extrude "Extrude2''" cut sketch "Sketch106" along normal up to surface (6.8 mm away) contours L0 L1 L3 L7 bodies 13 in component "Mechanism_backstop"